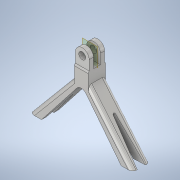
# Autodesk Inventor part: noga
Saved by Autodesk Inventor 2020 (Build 240168000, 168)
## iProperties
Created: 2019-11-17
Part Number: noga
Material: Ogólny
Document SubType Name: Modeling
Designer: macie
Density: 1 g/cm^3
Appearance: Domyślna
Author: macie
## iProperties of the stored document _Drukowanie 3D.ipt
Created: 2019-12-29
Part Number: _Drukowanie 3D
Material: Ogólny
Document SubType Name: Modeling
Designer: macie
Density: 1 g/cm^3
Appearance: Domyślna
Author: macie
Autodesk Inventor part; units mm, degrees
ref_plane "YZ Plane" through (0, 0, 0) normal (1, 0, 0) x (0, 1, 0)
ref_plane "XZ Plane" through (0, 0, 0) normal (0, 1, 0) x (-1, 0, 0)
ref_plane "XY Plane" through (0, 0, 0) normal (0, 0, 1) x (1, 0, 0)
sketch "Szkic1" plane through (0, 0, 0) normal (0, 0, 1) x (1, 0, 0)
  circle A0 centre (0, 0) radius 3
  arc A1 (6, 0) -> (-6, 0) centre (0, 0) ccw
  line L0 (-6, 0) -> (-6, -19)
  line L1 (6, 0) -> (6, -19)
  line L2 (6, -19) -> (44.5673, -64.9627)
  line L3 (44.5673, -64.9627) -> (34.5673, -64.9627)
  line L4 (34.5673, -64.9627) -> (0, -20.8894)
  line L5 (0, 0) -> (0, -6.4969) construction
  line L6 (-6, 0) -> (-6, -19)
  line L7 (-6, -19) -> (-44.5673, -64.9627)
  line L8 (-44.5673, -64.9627) -> (-34.5673, -64.9627)
  line L9 (-34.5673, -64.9627) -> (0, -20.8894)
  dimension "d0" = 6
  dimension "d1" = 12
  dimension "d2" = 19
  dimension "d3" = 19
  dimension "d4" = 60
  dimension "d5" = 140
  dimension "d6" = 10
  constraints: 20 end point, 2 centre point, 2 coincident, 2 point on circle, 2 symmetric about line, 2 vertical, 1 parallel, 1 perpendicular, 1 tangent
  measures "d0" diameter of A0
  measures "d1" diameter of A1
  measures "d2" distance of L0.start L0.end
  measures "d3" distance of L1.start L1.end
  measures "d4" distance of L1.end L2.end
  measures "d5" angle of L2 L1
  measures "d6" distance of L2.end L3.end
extrude "Wyciągnięcie proste1" add sketch "Szkic1" along normal blind 5
sketch "Szkic2" plane through (0, 0, 5) normal (0, 0, 1) x (1, 0, 0)
  circle A0 centre (0, 0) radius 3 construction
  line L0 (-6, 0) -> (-6, -19) construction
  line L1 (-6, -19) -> (-44.5673, -64.9627) projected
  line L2 (-44.5673, -64.9627) -> (-34.5673, -64.9627) projected
  line L3 (-34.5673, -64.9627) -> (0, -20.8894) projected
  line L4 (0, -20.8894) -> (34.5673, -64.9627) projected
  line L5 (34.5673, -64.9627) -> (44.5673, -64.9627) projected
  line L6 (44.5673, -64.9627) -> (6, -19) projected
  line L7 (6, -19) -> (6, 0) construction
  arc A1 (6, 0) -> (-6, 0) centre (0, 0) ccw construction
  line L8 (-6, 0) -> (-6, -19) construction
  line L9 (-6, -8.5404) -> (6, -8.5404)
  line L10 (-6, -19) -> (-6, -8.5404)
  line L11 (6, -19) -> (6, -8.5404)
  line L12 (6, -19) -> (6, 0) projected
  constraints: 6 end point, 2 collinear, 2 point on line, 1 perpendicular
extrude "Wyciągnięcie proste2" add sketch "Szkic2" along normal blind 5
sketch "Szkic3" plane through (0, 0, 10) normal (0, 0, 1) x (1, 0, 0)
  circle A0 centre (0, 0) radius 3 projected
  line L0 (-6, 0) -> (-6, -19) projected
  arc A1 (6, 0) -> (-6, 0) centre (0, 0) ccw projected
  line L1 (6, -19) -> (6, 0) projected
  line L2 (44.5673, -64.9627) -> (6, -19) projected
  line L3 (34.5673, -64.9627) -> (44.5673, -64.9627) projected
  line L4 (0, -20.8894) -> (34.5673, -64.9627) projected
  line L5 (-34.5673, -64.9627) -> (0, -20.8894) projected
  line L6 (-44.5673, -64.9627) -> (-34.5673, -64.9627) projected
  line L7 (-6, -19) -> (-44.5673, -64.9627) projected
extrude "Wyciągnięcie proste3" add sketch "Szkic3" along normal blind 5
sketch "Szkic4" plane through (-44.5673, -64.9627, 0) normal (-0.7660444, 0.6427876, 0) x (0, 0, 1)
  line L0 (0, 0) -> (15, 0) projected
  line L1 (11.054, 0) -> (7.5, 50.8667)
  line L2 (0, 50.8667) -> (15, 50.8667) projected
  line L3 (5, 68.0125) -> (10, 68.0125) construction
  line L4 (7.5, 68.0125) -> (7.5, 50.8667) construction
  line L5 (3.946, 0) -> (7.5, 50.8667)
  line L6 (3.946, 0) -> (11.054, 0)
  point P0 (0, 78.4116)
  constraints: 8 end point, 2 midpoint, 1 collinear, 1 point on line, 1 symmetric about line, 1 vertical
extrude "Wyciągnięcie proste4" cut sketch "Szkic4" against normal blind 25.75
mirror "Odbij1" about plane through (0, 0, 0) normal (1, 0, 0) of "Wyciągnięcie proste4"
fillet "Zaokrąglenie1" radius 5 1 edges at (0, -20.8894, 7.5)
fillet "Zaokrąglenie2" radius 1 1 edges at (9.4991, -27.9866, 7.5)
fillet "Zaokrąglenie3" radius 1 1 edges at (-9.4991, -27.9866, 7.5)
fillet "Zaokrąglenie4" radius 3 4 edges at (-25.2836, -41.9813, 0) (-25.2836, -41.9813, 15) (25.2836, -41.9813, 15) (25.2836, -41.9813, 0)
ref_plane "Płaszczyzna konstrukcyjna1" through (0, 0, 7.5) normal (0, 0, 1) x (1, 0, 0)
split "Podział1" plane through (0, 0, 7.5) removes the side toward (0, 0, 1)
mirror "Odbij2" about plane through (0, 0, 7.5) normal (0, 0, 1)
ref_plane "Płaszczyzna konstrukcyjna2" through (0, 0, 7.5) normal (0, 0, -1) x (-1, 0, 0)
sketch "Szkic6" plane through (0, 0, 7.5) normal (0, 0, -1) x (-1, 0, 0)
  line L0 (6, -8.5404) -> (-6, -8.5404) projected
  line L1 (6, -8.5404) -> (-12.1779, -8.5404)
  line L2 (-12.1779, -8.5404) -> (-12.1779, 12.1353)
  line L3 (-12.1779, 12.1353) -> (6, 12.1353)
  line L4 (6, 12.1353) -> (6, -8.5404)
  point P0 (0, 0)
  constraints: 8 end point, 2 parallel, 1 horizontal, 1 perpendicular
extrude "Wyciągnięcie proste5" cut sketch "Szkic6" along normal mid plane 6
sketch "Szkic7" plane through (0, 0, 15) normal (0, 0, 1) x (1, 0, 0)
  line L0 (6, -8.5404) -> (-6, -8.5404) projected
  line L1 (-6, -8.5404) -> (8.236, -8.5404)
  line L2 (8.236, -8.5404) -> (8.236, 11.1048)
  line L3 (8.236, 11.1048) -> (-6, 11.1048)
  line L4 (-6, 11.1048) -> (-6, -8.5404)
  point P0 (0, 0)
  constraints: 8 end point, 2 parallel, 1 horizontal, 1 perpendicular
extrude "Wyciągnięcie proste6" cut sketch "Szkic7" against normal blind 0.8
sketch "Szkic8" plane through (0, 0, 0) normal (0, 0, -1) x (-1, 0, 0)
  line L0 (-6, -8.5404) -> (6, -8.5404) projected
  line L1 (6, -8.5404) -> (-9.6334, -8.5404)
  line L2 (-9.6334, -8.5404) -> (-9.6334, 6.7857)
  line L3 (-9.6334, 6.7857) -> (6, 6.7857)
  line L4 (6, 6.7857) -> (6, -8.5404)
  point P0 (0, 0)
  constraints: 8 end point, 2 parallel, 1 horizontal, 1 perpendicular
extrude "Wyciągnięcie proste7" cut sketch "Szkic8" against normal blind 0.8
fillet "Zaokrąglenie5" radius 2 2 edges at (0, -8.5404, 15) (0, -8.5404, 0)
